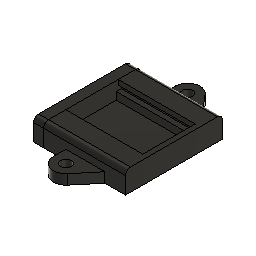
load cell amp buddy (Autodesk Fusion 360 design; units mm, degrees)
Autodesk Fusion 360 part; units mm, degrees
sketch "Sketch1" plane through (0, 0, 0) normal (1, 0, 0) x (0, 1, 0)
  circle A0 centre (-15.5, 2) radius 1.5
  line L0 (-19.5, 0) -> (-19.5, 4.8)
  line L1 (-17.5, 6.8) -> (-10.55, 6.8)
  line L2 (-10.55, 6.8) -> (-10.55, 4.8)
  line L3 (-10.55, 4.8) -> (-11.75, 4.8)
  line L4 (-11.75, 4.8) -> (-11.75, 3)
  line L5 (-11.75, 3) -> (-9.75, 3)
  line L6 (-9.75, 3) -> (-9.75, 0)
  line L7 (-9.75, 0) -> (0, 0)
  line L8 (0, 0) -> (0, -24.868) construction
  circle A1 centre (-15.5, 2) radius 2.75 construction
  arc A2 (-17.5, 6.8) -> (-19.5, 4.8) centre (-17.5, 4.8) ccw
  line L9 (-19.5, 0) -> (-19.5, -2)
  line L10 (-19.5, -2) -> (0, -2)
  line L11 (17.5, 6.8) -> (10.55, 6.8)
  line L12 (19.5, 0) -> (19.5, -2)
  circle A3 centre (15.5, 2) radius 1.5
  line L13 (11.75, 3) -> (9.75, 3)
  line L14 (9.75, 3) -> (9.75, 0)
  line L15 (11.75, 4.8) -> (11.75, 3)
  line L16 (19.5, 0) -> (19.5, 4.8)
  line L17 (19.5, -2) -> (0, -2)
  arc A4 (19.5, 4.8) -> (17.5, 6.8) centre (17.5, 4.8) ccw
  line L18 (10.55, 6.8) -> (10.55, 4.8)
  line L19 (9.75, 0) -> (0, 0)
  line L20 (10.55, 4.8) -> (11.75, 4.8)
  line L21 (19.5, 2) -> (11.5, 2) construction
  circle A5 centre (15.5, 2) radius 2.75 construction
  dimension "d1" = 5.5
  dimension "d2" = 3
  dimension "d5" = 11.75
  dimension "d8" = 2
  dimension "d9" = 1.2
  dimension "d10" = 2
  dimension "d11" = 3
  dimension "d12" = 1.8
  dimension "d14" = 2
  dimension "d19" = 2
  dimension "d32" = 19.5
  constraint vertical L0
  constraint perpendicular L0 L1
  constraint perpendicular L1 L2
  constraint perpendicular L2 L3
  constraint perpendicular L3 L4
  constraint perpendicular L4 L5
  constraint perpendicular L5 L6
  constraint perpendicular L6 L7
  constraint coincident L7.end L8.start
  constraint vertical L8
  constraint concentric A0 A1
  constraint coincident L7.end L8
  constraint tangent L1 A2
  constraint tangent L0 A2
  constraint coincident L0 L9.end
  constraint coincident L9.end L10.start
  constraint coincident L9.end L10
  constraint coincident L8 L10.end
  constraint horizontal L10
  constraint symmetric L7.end L8 L19.end
  constraint symmetric A0 L8 A3
  constraint symmetric L1.end L8 L11.end
  constraint symmetric L2.end L8 L18.end
  constraint symmetric L3.end L8 L15.start
  constraint symmetric L4.end L8 L13.start
  constraint symmetric L5.end L8 L13.end
  constraint symmetric L6.end L8 L14.end
  constraint symmetric L8 L9.end L12.end
  constraint symmetric L8 A1 A5
  constraint symmetric L8 L1.start L11.start
  constraint symmetric L8 L0.end L16.end
  constraint symmetric L8 A2 A4
  constraint symmetric L8 L0.start L12.start
  constraint symmetric L8 L10.end L17.end
  measures "d1" diameter of A1
  measures "d2" diameter of A0
  measures "d5" distance of L7.end L4
  measures "d8" distance of L4.end L5.end
  measures "d9" distance of L2.end L3.end
  measures "d10" distance of L1.end L2.end
  measures "d11" distance of L5.end L6.end
  measures "d12" distance of L3.end L4.end
  measures "d14" radius of A2
  measures "d19" distance of L7.end L10.end
  measures "d32" horizontal distance of L9.end L7.end
extrude "Extrude1" add sketch "Sketch1" along normal blind 31 makes body 1
sketch "Sketch2" plane through (31, 0, 0) normal (1, 0, 0) x (0, 1, 0)
  circle A0 centre (-15.5, 2) radius 1.5
  line L0 (9.75, 0) -> (-9.75, 0)
  line L1 (-9.75, 0) -> (-9.75, 3)
  line L2 (-9.75, 3) -> (-11.75, 3)
  line L3 (-11.75, 3) -> (-11.75, 4.8)
  line L4 (-11.75, 4.8) -> (-10.55, 4.8)
  line L5 (-10.55, 4.8) -> (-10.55, 6.8)
  line L6 (-10.55, 6.8) -> (-17.5, 6.8)
  arc A1 (-17.5, 6.8) -> (-19.5, 4.8) centre (-17.5, 4.8) ccw
  line L7 (-19.5, 4.8) -> (-19.5, -2)
  line L8 (-10.55, 6.8) -> (10.55, 6.8)
  line L9 (19.5, -2) -> (19.5, 4.8)
  arc A2 (19.5, 4.8) -> (17.5, 6.8) centre (17.5, 4.8) ccw
  line L10 (17.5, 6.8) -> (10.55, 6.8)
  line L11 (10.55, 6.8) -> (10.55, 4.8)
  line L12 (10.55, 4.8) -> (11.75, 4.8)
  line L13 (11.75, 4.8) -> (11.75, 3)
  line L14 (11.75, 3) -> (9.75, 3)
  line L15 (9.75, 3) -> (9.75, 0)
  line L16 (-19.5, -2) -> (19.5, -2)
  circle A3 centre (15.5, 2) radius 1.5
  constraint coincident L5.end L6.start
  constraint coincident L8.end L10.end
extrude "Extrude2" add sketch "Sketch2" along normal blind 2 contours A0 | L0 L1 L2 L3 L4 L5 L6 A1 L7 L9 A2 L10 L11 L12 L13 L14 L15 L16 | L0 L1 L2 L3 L4 L5 L8 L11 L12 L13 L14 L15 | A3 bodies 1
sketch "Sketch3" plane through (0, 0, -2) normal (0, 0, -1) x (1, 0, 0)
  line L0 (0, 19.5) -> (0, -19.5)
  line L1 (0, -19.5) -> (33, -19.5)
  line L2 (33, -19.5) -> (33, 19.5)
  line L3 (33, 19.5) -> (0, 19.5)
  line L4 (0, 0) -> (33, 0) construction
  circle A0 centre (14, 24.5) radius 2.1
  circle A1 centre (14, 24.5) radius 5
  line L5 (9, 24.5) -> (9, 19.5)
  line L6 (17.8302, 27.7139) -> (24.7225, 19.5)
  circle A2 centre (14, -24.5) radius 5
  circle A3 centre (14, -24.5) radius 2.1
  line L7 (17.8302, -27.7139) -> (24.7225, -19.5)
  line L8 (9, -24.5) -> (9, -19.5)
  point P0 (33, -19.5)
  point P1 (0, -19.5)
  point P2 (16.5, -24.5)
  dimension "d20" = 4.2
  dimension "d22" = 10
  dimension "d30" = 50
  dimension "d31" = 14
  constraint coincident L4.start origin
  constraint perpendicular L0 L4
  constraint coincident L2 L4.end
  constraint concentric A0 A1
  constraint coincident A1 L5.start
  constraint tangent A1 L5
  constraint coincident L3 L5.end
  constraint perpendicular L3 L5
  constraint tangent L3 A1
  constraint coincident L3 L6.end
  constraint tangent A1 L6
  constraint coincident A1 L6.start
  constraint symmetric L0.start L4 L0.end
  constraint symmetric L2.end L4 P0
  constraint symmetric L4 A0 A3
  constraint symmetric L4 A1 A2
  constraint symmetric L4 L5.start L8.start
  constraint symmetric L4 L5.end L8.end
  constraint symmetric L4 L6.start L7.start
  constraint symmetric L4 L6.end L7.end
  measures "d20" diameter of A0
  measures "d22" diameter of A1
  measures "d30" angle of L3 L6
  measures "d31" horizontal distance of L4.start A0.centre
extrude "Extrude3" add sketch "Sketch3" against normal blind 4 contours L3 A1 L5 | L1 A2 L8 | L3 A1 L6 | A1 | L1 A2 L7 | A2 bodies 1
sketch "Sketch1 (2)" plane through (0, 0, 0) normal (-1, 0, 0) x (0, -1, 0) in component "end cap"
  line L0 (-19.5, 4.8) -> (-19.5, -2)
  line L1 (-19.5, -2) -> (19.5, -2)
  line L2 (19.5, -2) -> (19.5, 4.8)
  arc A0 (19.5, 4.8) -> (17.5, 6.8) centre (17.5, 4.8) ccw
  line L3 (17.5, 6.8) -> (10.55, 6.8)
  line L4 (10.55, 6.8) -> (10.55, 4.8)
  line L5 (10.55, 4.8) -> (11.75, 4.8)
  line L6 (11.75, 4.8) -> (11.75, 3)
  line L7 (-9.75, 3) -> (-11.75, 3)
  line L8 (-11.75, 3) -> (-11.75, 4.8)
  line L9 (-11.75, 4.8) -> (-10.55, 4.8)
  line L10 (-10.55, 4.8) -> (-10.55, 6.8)
  line L11 (-10.55, 6.8) -> (-17.5, 6.8)
  arc A1 (-17.5, 6.8) -> (-19.5, 4.8) centre (-17.5, 4.8) ccw
  line L12 (-10.55, 6.8) -> (10.55, 6.8)
  circle A2 centre (-15.5, 2) radius 3
  circle A3 centre (15.5, 2) radius 3
  line L13 (-9.75, 0) -> (-9.75, 3)
  line L14 (11.75, 3) -> (9.75, 3)
  line L15 (9.75, 3) -> (9.75, 0)
  circle A4 centre (15.5, 2) radius 1.5
  circle A5 centre (-15.5, 2) radius 1.5
  line L16 (9.75, 0) -> (-9.75, 0)
  dimension "d27" = 6
  constraint coincident L10.end L11.start
  constraint coincident L3.end L4.start
  constraint concentric A2 A5
  constraint equal A2 A3
  measures "d27" diameter of A2
extrude "Extrude1'" add sketch "Sketch1 (2)" along normal blind 4 separate body contours L0 L1 L2 A0 L3 L4 L5 L6 L7 L8 L9 L10 L11 A1 L13 L14 L15 L16 | L4 L5 L6 L7 L8 L9 L10 L12 L13 L14 L15 L16 | A2 | A3 makes body 2 in component "end cap"
extrude "Extrude2'" cut sketch "Sketch1 (2)" along normal through all from surface at 2 contours A2 | A3 | A4 bodies 2 in component "end cap"
component "end cap" placed x (1, 0, 0) y (0, 1, 0) z (0, 0, 1) at (0, 0, 0)
equation "d5 = ( 23.5 / 2 ) * 1 mm"
named bodies: "load cell amp buddy base", "load cell amp end cap"
